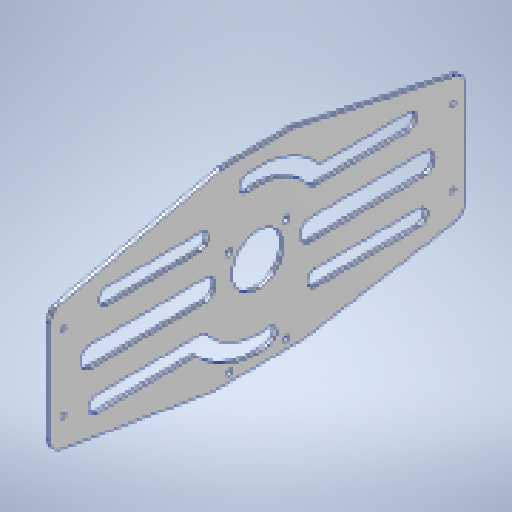
# Autodesk Inventor part: joint_adaptor_plate
Saved by Autodesk Inventor 2024 (Build 280153000, 153)
## iProperties
Created: 2025-06-28
Part Number: joint_adaptor_plate
Material: アルミニウム 6061
Document SubType Name: Sheet Metal
Designer: kshau
Density: 2.7 g/cm^3
Appearance: アルミニウム - フラット
Mass: 22.0785 g
Surface Area: 182.485 cm^2
Volume: 22.0785 cm^3
Sheet Metal Rule: Default
Author: kshau
Autodesk Inventor part; units mm, degrees
ref_plane "YZ Plane" through (0, 0, 0) normal (1, 0, 0) x (0, 1, 0)
ref_plane "XZ Plane" through (0, 0, 0) normal (0, 1, 0) x (-1, 0, 0)
ref_plane "XY Plane" through (0, 0, 0) normal (0, 0, 1) x (1, 0, 0)
sketch "スケッチ1" plane through (0, 0, 0) normal (1, 0, 0) x (0, 1, 0)
  line L0 (37.123, 0) -> (-35.25, 0)
  line L1 (-35.25, 0) -> (-35.25, -80)
  line L2 (-35.25, -80) -> (37.123, -80)
  line L3 (37.123, -80) -> (37.123, 0)
  line L4 (-35.25, 0) -> (-35.25, -17.883)
  line L5 (37.123, 0) -> (37.123, -13.85)
  line L6 (37.123, -13.85) -> (22.5, -80)
  line L7 (-35.25, -17.883) -> (-24.5, -80)
  circle A0 centre (0, 0) radius 9.85
  line L8 (0, 0) -> (0, -80)
  line L9 (14.5, -80) -> (0, -80)
  line L10 (0, -80) -> (0, -75)
  line L11 (0, -75) -> (14.5, -75)
  line L12 (14.5, -75) -> (14.5, -80)
  line L13 (0, -75) -> (-14.5, -75)
  line L14 (-14.5, -75) -> (-14.5, -80)
  circle A1 centre (0, -20.151) radius 4
  circle A2 centre (0, -64.253) radius 4
  line L15 (4, -20.151) -> (4, -64.253)
  line L16 (-4, -64.253) -> (-4, -20.151)
  line L17 (11.25, 0) -> (-35.25, 0)
  line L18 (-35.25, 0) -> (-35.25, -14.25)
  line L19 (-35.25, -14.25) -> (11.25, -14.25)
  line L20 (11.25, -14.25) -> (11.25, 0)
  circle A3 centre (17, -22.151) radius 3.1
  line L21 (17, -22.151) -> (17, -58.151)
  circle A4 centre (17, -58.151) radius 3.1
  line L22 (20.1, -22.151) -> (20.1, -58.151)
  line L23 (13.9, -58.151) -> (13.9, -22.151)
  circle A5 centre (-17, -22.151) radius 3.1
  line L24 (-17, -22.151) -> (-17, -62.151)
  circle A6 centre (-17, -62.151) radius 3.1
  line L25 (-13.9, -22.151) -> (-13.9, -62.151)
  line L26 (-20.1, -22.151) -> (-20.1, -62.151)
  line L27 (-35.25, 0) -> (-35.25, 80)
  line L28 (-35.25, 80) -> (37.123, 80)
  line L29 (37.123, 80) -> (37.123, 0)
  line L30 (-35.25, 0) -> (-35.25, 17.883)
  line L31 (37.123, 0) -> (37.123, 13.85)
  line L32 (37.123, 13.85) -> (22.5, 80)
  line L33 (-35.25, 17.883) -> (-24.5, 80)
  circle A7 centre (0, 20.151) radius 4
  circle A8 centre (0, 64.253) radius 4
  line L34 (4, 20.151) -> (4, 64.253)
  line L35 (-4, 64.253) -> (-4, 20.151)
  circle A9 centre (17, 22.151) radius 3.1
  line L36 (17, 22.151) -> (17, 58.151)
  circle A10 centre (17, 58.151) radius 3.1
  line L37 (20.1, 22.151) -> (20.1, 58.151)
  line L38 (13.9, 58.151) -> (13.9, 22.151)
  circle A11 centre (-17, 22.151) radius 3.1
  circle A12 centre (-17, 62.151) radius 3.1
  line L39 (-13.9, 22.151) -> (-13.9, 62.151)
  line L40 (-20.1, 22.151) -> (-20.1, 62.151)
  dimension "d0" = 72.373
  dimension "d1" = 37.123
  dimension "d2" = 80
  dimension "d3" = 17.883
  dimension "d4" = 13.85
  dimension "d7" = 19.7
  dimension "d8" = 14.5
  dimension "d9" = 5
  dimension "d10" = 8
  dimension "d11" = 10
  dimension "d12" = 8
  dimension "d13" = 20.151
  dimension "d14" = 8
  dimension "d15" = 15.747
  dimension "d16" = 11.25
  dimension "d17" = 14.25
  dimension "d18" = 6.2
  dimension "d19" = 17
  dimension "d20" = 22.151
  dimension "d21" = 36
  dimension "d22" = 6.2
  dimension "d23" = 6.2
  dimension "d24" = 22.151
  dimension "d25" = 17
  dimension "d26" = 40
  dimension "d27" = 6.2
  constraints: 82 end point, 27 symmetric about line, 24 point on circle, 16 point on line, 13 centre point, 12 tangent, 6 parallel, 4 coincident, 4 perpendicular, 3 horizontal, 2 vertical, 6 other
  measures "d0" distance of L1.end L2.end
  measures "d1" distance from line of point (0, 0) L3
  measures "d2" distance of L2.end L0.start
  measures "d3" distance of L0.end L4.end
  measures "d4" distance of L0.start L5.end
  measures "d7" diameter of A0
  measures "d8" distance of L10.end L11.end
  measures "d9" distance of L11.end L9.start
  measures "d10" distance from line of L12 L6.end
  measures "d11" distance from line of L14 L7.end
  measures "d12" diameter of A1
  measures "d13" distance of L8.start A1.centre
  measures "d14" diameter of A2
  measures "d15" distance from line of L2 A2.centre
  measures "d16" distance from line of L8.start L20
  measures "d17" distance from line of L8.start L19
  measures "d18" diameter of A3
  measures "d19" distance from line of L8 L21.start
  measures "d20" distance from line of L0 L21.start
  measures "d21" distance of L21.start L21.end
  measures "d22" diameter of A4
  measures "d23" diameter of A5
  measures "d24" distance from line of L0 L24.start
  measures "d25" distance from line of L8 L24.start
  measures "d26" distance of L24.start L24.end
  measures "d27" diameter of A6
extrude "押し出し1" add sketch "スケッチ1" along normal blind 1.5 contours L3 L6 L2 L12 L11 L8 A2 L15 A1 L19 L20 L0 | L0 A0 L27 L33 L28 L32 L29 | L20 L19 L8 A0 L0 | A0 L8 L19 L1 L0 | L8 A1 L16 A2 L13 L14 L2 L7 L1 L19 | L2 L8 L11 L12 | L2 L14 L13 L8
sketch "スケッチ2" plane through (1.5, 0, 0) normal (1, 0, 0) x (0, 0, -1)
  line L0 (-17.883, -35.25) -> (17.883, -35.25) projected
  line L1 (0, 11.25) -> (14.25, 11.25)
  line L2 (14.25, 11.25) -> (14.25, -35.25)
  line L3 (14.25, -35.25) -> (0, -35.25)
  line L4 (0, -35.25) -> (0, 11.25)
  circle A0 centre (0, 0) radius 9.85 projected
  point P0 (11, 8)
  point P1 (11, -32)
  point P2 (-11, 8)
  point P3 (-11, -32)
  dimension "d30" = 14.25
  dimension "d31" = 11.25
  dimension "d32" = 3.25
  dimension "d33" = 3.25
  dimension "d34" = 3.25
  dimension "d35" = 3.25
  constraints: 8 end point, 2 parallel, 2 point on line, 2 symmetric about line, 1 horizontal, 1 perpendicular
  measures "d30" distance of L1.start L1.end
  measures "d31" distance from line of A0.centre L1
  measures "d32" distance from line of L1 point (11, 8)
  measures "d33" distance from line of L2 point (11, 8)
  measures "d34" distance from line of L2 point (11, -32)
  measures "d35" distance from line of L0 point (11, -32)
hole "穴1" at (1.5, 8, -11) at (1.5, -32, -11) at (1.5, 8, 11) at (1.5, -32, 11) direction (-1, 0, 0) diameter 2.5 end through all
sketch "スケッチ3" plane through (1.5, 0, 0) normal (1, 0, 0) x (0, 0, -1)
  line L0 (0, 0) -> (80, 0)
  line L1 (80, -24.5) -> (80, 22.5) projected
  line L2 (13.85, 37.123) -> (-13.85, 37.123) projected
  line L3 (0, 37.123) -> (0, -35.25)
  line L4 (-17.883, -35.25) -> (17.883, -35.25) projected
  point P0 (75, 14.5)
  point P1 (75, -14.5)
  point P2 (-75, 14.5)
  point P3 (-75, -14.5)
  dimension "d43" = 5
  dimension "d44" = 14.5
  constraints: 4 end point, 3 symmetric about line, 2 midpoint, 1 horizontal, 1 point on line
  measures "d43" distance from line of L1 point (75, 14.5)
  measures "d44" distance from line of L0 point (75, 14.5)
hole "穴2" at (1.5, 14.5, -75) at (1.5, -14.5, -75) at (1.5, 14.5, 75) at (1.5, -14.5, 75) direction (-1, 0, 0) diameter 2.1 end through all
fillet "フィレット1" radius 5 4 edges at (0.75, 22.5, -80) (0.75, -24.5, -80) (0.75, 22.5, 80) (0.75, -24.5, 80)
sketch "スケッチ4" plane through (0, 0, 0) normal (-1, 0, 0) x (0, 0, 1)
  circle A0 centre (0, 0) radius 27.5
  arc A1 (-22.151, 13.9) -> (-22.151, 20.1) centre (-22.151, 17) ccw projected
  circle A2 centre (-22.151, 17) radius 3.1
  arc A3 (22.151, -13.9) -> (22.151, -20.1) centre (22.151, -17) ccw projected
  circle A4 centre (22.151, -17) radius 3.1
  arc A5 (-22.151, -20.1) -> (-22.151, -13.9) centre (-22.151, -17) ccw projected
  circle A6 centre (-22.151, -17) radius 3.1
  arc A7 (22.151, 20.1) -> (22.151, 13.9) centre (22.151, 17) ccw projected
  circle A8 centre (22.151, 17) radius 3.1
  circle A9 centre (0, 0) radius 24.8225
  circle A10 centre (0, 0) radius 31.0225
  line L0 (0, 0) -> (8.0292, 29.9654)
  line L1 (0, 0) -> (0, 31.0225)
  line L2 (0, 0) -> (-8.0292, -29.9654)
  circle A11 centre (7.2269, 26.9711) radius 3.1
  circle A12 centre (-7.2269, -26.9711) radius 3.1
  line L3 (0, 0) -> (13.1107, -28.1159)
  circle A13 centre (11.8006, -25.3064) radius 3.1
  line L4 (0, 0) -> (-13.1107, 28.1159)
  circle A14 centre (-11.8006, 25.3064) radius 3.1
  point P0 (19.6918, -15.1126)
  point P1 (-19.6918, -15.1126)
  point P2 (-24.6102, -18.8874)
  point P3 (24.6102, -18.8874)
  point P4 (24.6102, 18.8874)
  point P5 (-24.6102, 18.8874)
  point P6 (-22.151, 20.1)
  point P7 (-19.6918, 15.1126)
  point P8 (19.6918, 15.1126)
  point P9 (22.151, 20.1)
  point P10 (-8.0292, -29.9654)
  point P11 (-6.4245, -23.9767)
  point P12 (8.0292, 29.9654)
  point P13 (6.4245, 23.9767)
  point P14 (10.4904, -22.4968)
  point P15 (-10.4904, 22.4968)
  dimension "d53" = 55
  dimension "d56" = 15
  dimension "d57" = 25
  constraints: 10 end point, 8 tangent, 7 centre point, 7 coincident, 5 point on circle, 4 point on line, 2 collinear, 1 vertical, 14 other
  measures "d53" diameter of A0
  measures "d56" angle of L1 L0
  measures "d57" angle of L1 L3
extrude "押し出し2" cut sketch "スケッチ4" against normal blind 10 contours A4 A3 A0 | A0 A3 A4 | A3 A4 A10 A13 A0 | A0 A13 A9 A3 | A13 L3 A0 | A0 L3 A13 | L3 A13 A0 | A0 A13 L3 | A14 A0 L4 | A9 A1 A0 A14 | L4 A0 A14 | A14 A0 A1 A2 A10 | A14 A0 L4 | L4 A0 A14 | A1 A2 A0 | A2 A1 A0
equation "\"BendRadius\" = Thickness"
equation "\"BendReliefWidth\" = Thickness"
equation "\"BendReliefDepth\" = 0.5 * Thickness"
equation "\"CornerReliefSize\" = 4 * Thickness"
equation "\"MinimumRemnant\" = 2 * Thickness"
equation "\"TransitionRadius\" = BendRadius"
equation "\"JacobiRadiusSize\" = BendRadius"
equation "\"GapSize\" = Thickness"
equation "\"Thickness\" = 3.048"
